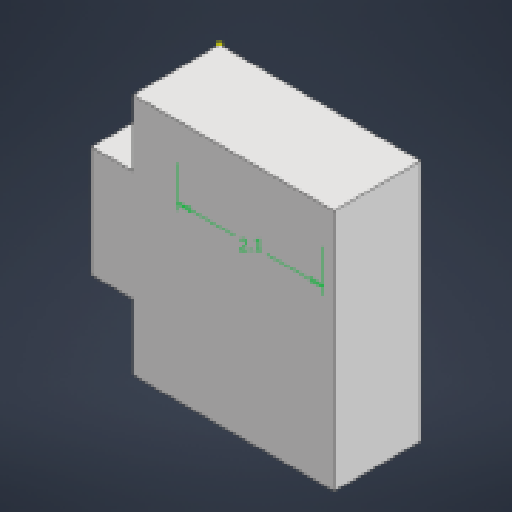
# Autodesk Inventor part: SKSCPAE010
Saved by Autodesk Inventor 2023 (Build 270158000, 158)
## iProperties
Created: 2022-10-25
Part Number: SKSCPAE010
Material: Generic
Document SubType Name: Modeling
Designer: jevan
Density: 1 g/cm^3
Appearance: Default
Author: jevan
Autodesk Inventor part; units mm, degrees
ref_plane "YZ Plane" through (0, 0, 0) normal (1, 0, 0) x (0, 1, 0)
ref_plane "XZ Plane" through (0, 0, 0) normal (0, 1, 0) x (-1, 0, 0)
ref_plane "XY Plane" through (0, 0, 0) normal (0, 0, 1) x (1, 0, 0)
sketch "Sketch1" plane through (0, 0, 0) normal (0, 0, 1) x (1, 0, 0)
  line L0 (0, 0) -> (2.9, 0)
  line L1 (2.9, 0) -> (2.9, -3.5)
  line L2 (2.9, -3.5) -> (0, -3.5)
  line L3 (0, -3.5) -> (0, 0)
  dimension "d0" = 2.9
  dimension "d1" = 3.5
  constraints: 8 end point, 2 parallel, 1 horizontal, 1 perpendicular
  measures "d0" distance of L1.end L2.end
  measures "d1" distance of L0.end L1.end
extrude "Extrusion1" add sketch "Sketch1" along normal blind 1.25
sketch "Sketch2" plane through (0, -3.5, 0) normal (-1, 0, 0) x (0, 0, 1)
  line L0 (1.25, 0) -> (1.25, 3.5) projected
  line L1 (1.25, 1.75) -> (0.15, 1.75)
  line L2 (0.15, 1.75) -> (0.15, 0.95)
  line L3 (0.15, 0.95) -> (1.25, 0.95)
  line L4 (1.25, 0.95) -> (1.25, 2.55)
  line L5 (1.25, 2.55) -> (0.15, 2.55)
  line L6 (0.15, 2.55) -> (0.15, 1.75)
  point P0 (0, 3.5)
  dimension "d4" = 1.1
  dimension "d5" = 0.8
  dimension "d6" = 1.6
  constraints: 12 end point, 5 perpendicular, 2 point on line, 1 horizontal, 1 midpoint
  measures "d4" distance of L1.start L1.end
  measures "d5" distance of L1.end L2.end
  measures "d6" distance of L3.end L4.end
extrude "Extrusion2" add sketch "Sketch2" along normal blind 0.6
sketch "Sketch3" plane through (0, 0, 0) normal (0, 0, -1) x (-1, 0, 0)
  line L0 (0.6, -2.55) -> (0.6, -0.95) projected
  line L1 (0.6, -1.75) -> (-1.5, -1.75)
  line L2 (-1.5, -1.75) -> (-1.5, -3.5)
  line L3 (0, -3.5) -> (-2.9, -3.5) projected
  line L4 (-1.5, -1.75) -> (-1.5, 0)
  line L5 (-2.9, 0) -> (0, 0) projected
  line L6 (-1.5, 0) -> (-0.85, 0)
  line L7 (-1.5, 0) -> (-2.15, 0)
  line L8 (-0.85, 0) -> (-0.5, 0)
  line L9 (-0.5, 0) -> (-0.5, 0.675)
  line L10 (-0.5, 0.675) -> (-1.2, 0.675)
  line L11 (-1.2, 0.675) -> (-1.2, 0)
  line L12 (-0.1, 0) -> (-3, 0)
  line L13 (-2.15, 0) -> (-2.5, 0)
  line L14 (-2.5, 0) -> (-2.5, 0.675)
  line L15 (-2.5, 0.675) -> (-1.8, 0.675)
  line L16 (-1.8, 0.675) -> (-1.8, 0)
  line L17 (-1.5, -3.5) -> (-0.85, -3.5)
  line L18 (-1.5, -3.5) -> (-2.15, -3.5)
  line L19 (-0.85, -3.5) -> (-0.5, -3.5)
  line L20 (-0.5, -3.5) -> (-0.5, -4.175)
  line L21 (-0.5, -4.175) -> (-1.2, -4.175)
  line L22 (-1.2, -4.175) -> (-1.2, -3.5)
  line L23 (-2.15, -3.5) -> (-2.5, -3.5)
  line L24 (-2.5, -3.5) -> (-2.5, -4.175)
  line L25 (-1.8, -4.175) -> (-1.8, -3.5)
  line L26 (-2.5, -4.175) -> (-1.8, -4.175)
  point P0 (-1.2, 0)
  point P1 (-1.8, 0)
  dimension "d9" = 2.1
  dimension "d10" = 0.65
  dimension "d11" = 0.65
  dimension "d12" = 0.35
  dimension "d13" = 0.675
  dimension "d14" = 0.7
  constraints: 48 end point, 16 symmetric about line, 8 point on line, 4 perpendicular, 1 horizontal, 1 midpoint, 1 vertical
  measures "d9" distance of L1.start L1.end
  measures "d10" distance of L4.end L6.end
  measures "d11" distance of L4.end L7.end
  measures "d12" distance of L6.end L8.end
  measures "d13" distance of L8.end L9.end
  measures "d14" distance of L9.end L10.end
extrude "Extrusion3" add sketch "Sketch3" against normal blind 0.1
body "Solid1"
